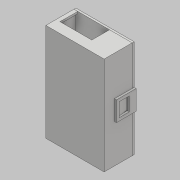
# Autodesk Inventor part: TTL-RS232transreceiverCover
Saved by Autodesk Inventor 2018 (Build 220112000, 112)
## iProperties
Created: 2019-07-02
Part Number: TTL-RS232transreceiverCover
Material: Generic
Document SubType Name: Modeling
Designer: mkivekas
Density: 1 g/cm^3
Appearance: Default
Author: mkivekas
Autodesk Inventor part; units mm, degrees
ref_plane "YZ Plane" through (0, 0, 0) normal (1, 0, 0) x (0, 1, 0)
sketch "Sketch1" plane through (0, 0, 0) normal (0, 1, 0) x (-1, 0, 0)
  line L0 (11.8161, 14.0771) -> (-17.6839, 14.0771)
  line L1 (-17.6839, 14.0771) -> (-17.6839, -35.4229)
  line L2 (-17.6839, -35.4229) -> (11.8161, -35.4229)
  line L3 (11.8161, -35.4229) -> (11.8161, 14.0771)
  point P0 (0, 0)
  dimension "d0" = 29.5
  dimension "d1" = 49.5
  constraints: 8 end point, 2 parallel, 1 horizontal, 1 perpendicular
  measures "d0" distance of L0.start L0.end
  measures "d1" distance of L2.end L0.start
extrude "Extrusion1" add sketch "Sketch1" along normal blind 1
sketch "Sketch2" plane through (0, 1, 0) normal (0, 1, 0) x (1, 0, 0)
  line L0 (-10.8161, -13.0771) -> (16.6839, -13.0771)
  line L1 (16.6839, -13.0771) -> (16.6839, 34.4229)
  line L2 (16.6839, 34.4229) -> (-10.8161, 34.4229)
  line L3 (-10.8161, 34.4229) -> (-10.8161, -13.0771)
  line L4 (-11.8161, 35.4229) -> (-11.8161, -14.0771) projected
  line L5 (17.6839, 35.4229) -> (-11.8161, 35.4229) projected
  line L6 (17.6839, -14.0771) -> (17.6839, 35.4229) projected
  line L7 (-11.8161, -14.0771) -> (17.6839, -14.0771) projected
  point P0 (0, 0)
  dimension "d4" = 1
  dimension "d5" = 1
  dimension "d6" = 1
  dimension "d7" = 1
  constraints: 8 end point, 2 parallel, 1 horizontal, 1 perpendicular
  measures "d4" distance between parallel lines of L4 L3
  measures "d5" distance between parallel lines of L5 L2
  measures "d6" distance between parallel lines of L6 L1
  measures "d7" distance between parallel lines of L7 L0
extrude "Extrusion2" add sketch "Sketch2" along normal blind 4.2
sketch "Sketch3" plane through (0, 5.2, 0) normal (0, 1, 0) x (1, 0, 0)
  line L0 (-11.8161, -14.0771) -> (17.6839, -14.0771) projected
  line L1 (-10.8161, -13.0771) -> (16.6839, -13.0771) projected
  line L2 (-9.8661, -14.0771) -> (6.2339, -14.0771)
  line L3 (6.2339, -14.0771) -> (6.2339, -13.0771)
  line L4 (6.2339, -13.0771) -> (-9.8661, -13.0771)
  line L5 (-9.8661, -13.0771) -> (-9.8661, -14.0771)
  line L6 (16.6839, 34.4229) -> (-10.8161, 34.4229) projected
  line L7 (17.6839, 35.4229) -> (-11.8161, 35.4229) projected
  line L8 (-10.1661, 34.4229) -> (5.9339, 34.4229)
  line L9 (5.9339, 34.4229) -> (5.9339, 35.4229)
  line L10 (5.9339, 35.4229) -> (-10.1661, 35.4229)
  line L11 (-10.1661, 35.4229) -> (-10.1661, 34.4229)
  line L12 (-11.8161, -14.0771) -> (17.6839, -14.0771)
  line L13 (17.6839, -14.0771) -> (17.6839, 35.4229)
  line L14 (17.6839, 35.4229) -> (-11.8161, 35.4229)
  line L15 (-11.8161, 35.4229) -> (-11.8161, -14.0771)
  line L16 (-10.8161, -13.0771) -> (16.6839, -13.0771)
  line L17 (16.6839, -13.0771) -> (16.6839, 34.4229)
  line L18 (16.6839, 34.4229) -> (-10.8161, 34.4229)
  line L19 (-10.8161, 34.4229) -> (-10.8161, -13.0771)
  point P0 (0, 0)
  dimension "d10" = 0.95
  dimension "d11" = 16.1
  dimension "d12" = 0.65
  dimension "d13" = 16.1
  constraints: 32 end point, 8 parallel, 4 horizontal, 4 perpendicular, 4 point on line
  measures "d10" distance from line of L5 L1.start
  measures "d11" distance between parallel lines of L5 L3
  measures "d12" distance from line of L11 L6.end
  measures "d13" distance between parallel lines of L11 L9
extrude "Extrusion3" add sketch "Sketch3" along normal blind 9 contours L15 L7 L11 L6 L19 L1 L5 L0 | L3 L1 L17 L6 L9 L7 L13 L0
sketch "Sketch4" plane through (0, 14.2, 0) normal (0, 1, 0) x (1, 0, 0)
  line L0 (-11.8161, 35.4229) -> (-11.8161, -14.0771) projected
  line L1 (-11.8161, -14.0771) -> (17.6839, -14.0771)
  line L2 (17.6839, -14.0771) -> (17.6839, 35.4229)
  line L3 (17.6839, 35.4229) -> (-11.8161, 35.4229)
  line L4 (-11.8161, 35.4229) -> (-11.8161, -14.0771)
  point P0 (0, 0)
  constraints: 8 end point, 2 parallel, 1 horizontal, 1 perpendicular
extrude "Extrusion4" add sketch "Sketch4" along normal blind 1 separate body
sketch "Sketch5" plane through (17.6839, 14.2, 14.0771) normal (1, 0, 0) x (0, 0, -1)
  line L0 (0, 1) -> (49.5, 1) projected
  line L1 (48.5, 0) -> (1, 0) projected
  line L2 (20, 1) -> (30, 1)
  line L3 (30, 1) -> (30, 0)
  line L4 (30, 0) -> (20, 0)
  line L5 (20, 0) -> (20, 1)
  line L6 (20, 0) -> (30, 0)
  line L7 (30, 0) -> (30, -9)
  line L8 (30, -9) -> (20, -9)
  line L9 (20, -9) -> (20, 0)
  point P0 (14.0771, -14.2)
  dimension "d18" = 10
  dimension "d19" = 20
  dimension "d20" = 9
  constraints: 16 end point, 4 parallel, 2 horizontal, 2 perpendicular, 2 point on line
  measures "d18" distance between parallel lines of L3 L5
  measures "d19" distance from line of L0.start L5
  measures "d20" distance of L6.end L7.end
extrude "Extrusion5" add sketch "Sketch5" along normal blind 1 bodies 2
sketch "Sketch6" plane through (-11.8161, 14.2, -35.4229) normal (-1, 0, 0) x (0, 0, 1)
  line L0 (0, 1) -> (49.5, 1) projected
  line L1 (19.5, -9) -> (19.5, 1) projected
  line L2 (29.5, 1) -> (19.5, 1)
  line L3 (19.5, 1) -> (19.5, -9)
  line L4 (19.5, -9) -> (29.5, -9)
  line L5 (29.5, -9) -> (29.5, 1)
  line L6 (49.5, 0) -> (49.5, 1) projected
  point P0 (35.4229, -14.2)
  dimension "d23" = 20
  constraints: 8 end point, 2 parallel, 1 horizontal, 1 perpendicular, 1 point on line
  measures "d23" distance between parallel lines of L6 L5
extrude "Extrusion6" add sketch "Sketch6" along normal blind 1 bodies 2
sketch "Sketch7" plane through (-12.8161, 14.2, -35.4229) normal (-1, 0, 0) x (0, 0, 1)
  line L0 (21, -7.5) -> (28, -7.5)
  line L1 (28, -7.5) -> (28, -2.5)
  line L2 (28, -2.5) -> (21, -2.5)
  line L3 (21, -2.5) -> (21, -7.5)
  line L4 (19.5, -9) -> (29.5, -9) projected
  line L5 (29.5, -9) -> (29.5, 1) projected
  line L6 (19.5, 1) -> (19.5, -9) projected
  point P0 (35.4229, -14.2)
  dimension "d26" = 1.5
  dimension "d27" = 1.5
  dimension "d28" = 1.5
  dimension "d29" = 5
  constraints: 8 end point, 2 parallel, 1 horizontal, 1 perpendicular
  measures "d26" distance between parallel lines of L4 L0
  measures "d27" distance between parallel lines of L5 L1
  measures "d28" distance between parallel lines of L6 L3
  measures "d29" distance of L0.end L1.end
extrude "Extrusion7" cut sketch "Sketch7" against normal blind 100 bodies 2
sketch "Sketch8" plane through (-11.8161, 0, -35.4229) normal (-1, 0, 0) x (0, 0, 1)
  line L0 (21.3, 11.4) -> (27.7, 11.4)
  line L1 (27.7, 11.4) -> (27.7, 7)
  line L2 (27.7, 7) -> (21.3, 7)
  line L3 (21.3, 7) -> (21.3, 11.4)
  line L4 (28, 11.7) -> (28, 6.7) projected
  line L5 (21, 6.7) -> (21, 11.7) projected
  line L6 (28, 6.7) -> (21, 6.7) projected
  line L7 (21, 11.7) -> (28, 11.7) projected
  point P0 (35.4229, 0)
  dimension "d32" = 0.3
  dimension "d33" = 0.3
  dimension "d34" = 0.3
  dimension "d35" = 0.3
  constraints: 8 end point, 2 parallel, 1 horizontal, 1 perpendicular
  measures "d32" distance between parallel lines of L4 L1
  measures "d33" distance between parallel lines of L5 L3
  measures "d34" distance between parallel lines of L6 L2
  measures "d35" distance between parallel lines of L0 L7
extrude "Extrusion8" add sketch "Sketch8" along normal blind 0.6 contours L0 L1 L2 L3 bodies 1
ref_plane "Work Plane1" through (-12.4161, 7, -7.7229) normal (0.9908, -0.1351, 0) x (0, 0, -1)
sketch "Sketch9" plane through (-12.4161, 7, -7.7229) normal (0.9908, -0.1351, 0) x (0, 0, -1)
  line L0 (6.4, 4.4407) -> (0, 4.4407) projected
  line L1 (6.4, 4.4407) -> (0, 4.4407)
  line L2 (0, 4.4407) -> (0, 0.003)
  line L3 (0, 0.003) -> (6.4, 0.003)
  line L4 (6.4, 0.003) -> (6.4, 4.4407)
  point P0 (-7.7229, -5.2582)
  constraints: 8 end point, 2 parallel, 1 horizontal, 1 perpendicular
extrude "Extrusion9" cut sketch "Sketch9" against normal blind 0.6 bodies 1
sketch "Sketch10" plane through (17.6839, 0, 14.0771) normal (1, 0, 0) x (0, 0, -1)
  line L0 (21.8, 11.4) -> (21.8, 7) projected
  line L1 (21.8, 7) -> (28.2, 7) projected
  line L2 (21.8, 11.4) -> (28.2, 11.4)
  line L3 (28.2, 11.4) -> (28.2, 7)
  line L4 (28.2, 7) -> (21.8, 7)
  line L5 (21.8, 7) -> (21.8, 11.4)
  point P0 (14.0771, 0)
  constraints: 8 end point, 2 parallel, 1 horizontal, 1 perpendicular
extrude "Extrusion10" add sketch "Sketch10" along normal blind 0.6 bodies 1
ref_plane "Work Plane2" through (18.2839, 7, -14.1229) normal (-0.9908, -0.1351, 0) x (0, 0, 1)
sketch "Sketch11" plane through (18.2839, 7, -14.1229) normal (-0.9908, -0.1351, 0) x (0, 0, 1)
  line L0 (6.4, 0.0811) -> (6.4, 4.4407) projected
  line L1 (6.4, 4.4407) -> (0, 4.4407)
  line L2 (0, 4.4407) -> (0, 0)
  line L3 (0, 0) -> (6.4, 0)
  line L4 (6.4, 0) -> (6.4, 4.4407)
  point P0 (14.1229, -4.4654)
  constraints: 8 end point, 2 parallel, 1 horizontal, 1 perpendicular
extrude "Extrusion11" cut sketch "Sketch11" against normal blind 0.6 bodies 1
body "Solid1"
body "Solid2"
